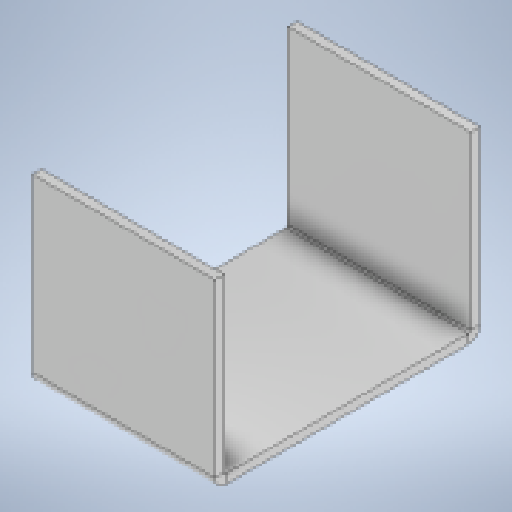
# Autodesk Inventor part: HWFrame
Saved by Autodesk Inventor 2025.2 (Build 292293000, 293)
## iProperties
Created: 2025-03-25
Part Number: HWFrame
Material: Aluminum 6061-AHC
Document SubType Name: Sheet Metal
Designer: User
Density: 2.7 g/cm^3
Sheet Metal Rule: Default_mm
Appearance: Aluminum - Dark
Author: User
Autodesk Inventor part; units mm, degrees
ref_plane "YZ Plane" through (0, 0, 0) normal (1, 0, 0) x (0, 1, 0)
ref_plane "XZ Plane" through (0, 0, 0) normal (0, 1, 0) x (-1, 0, 0)
ref_plane "XY Plane" through (0, 0, 0) normal (0, 0, 1) x (1, 0, 0)
sketch "Sketch1" plane through (0, 0, 0) normal (0, 1, 0) x (-1, 0, 0)
  line L0 (15, 20.25) -> (-15, 20.25)
  line L1 (-15, 20.25) -> (-15, -20.25)
  line L2 (-15, -20.25) -> (15, -20.25)
  line L3 (15, -20.25) -> (15, 20.25)
  line L4 (15, 20.25) -> (-15, -20.25) construction
  line L5 (-15, 20.25) -> (15, -20.25) construction
  point P0 (0, 0)
  dimension "d0" = 30
  dimension "d1" = 40.5
  measures "d0" distance of L1.end L2.end
  measures "d1" distance of L0.end L1.end
extrude "Plate1" add sketch "Sketch1" along normal blind 1.5
sketch "Sketch2" plane through (15, 0, 21.75) normal (0, 0, -1) x (-1, 0, 0)
  line L0 (30, 0) -> (0, 0)
  line L1 (0, 0) -> (0, 30)
  line L2 (0, 30) -> (30, 30)
  line L3 (30, 30) -> (30, 0)
  constraints: 8 end point
edge flange "Flange1" height 30 angle 90 thickness 1.5 bend radius 0.31 thickness toward (0, 0, -1) relief tear relief width 1.5 relief depth 0.75 corner gap 0.31 corner form 0 edges at (0, 1.5, 20.25) (0, 1.5, -20.25) wall of the first edge with corners at (-15, 0, 21.75) (15, 0, 21.75) (15, 30, 21.75) (-15, 30, 21.75)
bend "Bend1"
corner "Corner1"
sketch "Sketch3" plane through (-15, 30, 21.75) normal (0, 0, 1) x (1, 0, 0)
  circle A0 centre (22.525, -21) radius 0.7835 projected
  circle A1 centre (22.525, -5.9) radius 0.7835 projected
  circle A2 centre (7.475, -21) radius 0.7835 projected
  circle A3 centre (7.475, -5.9) radius 0.7835 projected
  ellipse E0 centre (22.952, 14.482) end of major axis (23.818, 15.348) minor radius 1 (24.07, 14.7056) -> (23.1756, 15.6) ccw projected
  line L0 (6.8244, 15.6) -> (23.1756, 15.6) projected
  ellipse E1 centre (7.048, 14.482) end of major axis (6.182, 15.348) minor radius 1 (6.8244, 15.6) -> (5.93, 14.7056) ccw projected
  line L1 (5.93, -21.6056) -> (5.93, 14.7056) projected
  ellipse E2 centre (7.048, -21.382) end of major axis (6.182, -22.248) minor radius 1 (5.93, -21.6056) -> (6.8244, -22.5) ccw projected
  line L2 (23.1756, -22.5) -> (6.8244, -22.5) projected
  ellipse E3 centre (22.952, -21.382) end of major axis (23.818, -22.248) minor radius 1 (23.1756, -22.5) -> (24.07, -21.6056) ccw projected
  line L3 (24.07, 14.7056) -> (24.07, -21.6056) projected
  circle A4 centre (7.475, -21) radius 0.7835 projected
  circle A5 centre (22.525, -21) radius 0.7835 projected
  circle A6 centre (7.475, -5.9) radius 0.7835 projected
  circle A7 centre (22.525, -5.9) radius 0.7835 projected
  circle A8 centre (7.475, 14.1) radius 0.7835 projected
  circle A9 centre (22.525, 14.1) radius 0.7835 projected
  circle A10 centre (15, 6.6) radius 6.4 projected
  point P0 (15, -30)
  constraints: 4 other
hole "Hole1" at (7.525, 24.1, 21.75) at (7.525, 9, 21.75) at (-7.525, 9, 21.75) at (-7.525, 24.1, 21.75) direction (0, 0, -1) diameter 2.1 depth 1.5
sketch "Sketch4" plane through (15, 30, -21.75) normal (0, 0, -1) x (-1, 0, 0)
  circle A0 centre (15, -20.82) radius 0.7835 projected
  circle A1 centre (8, -13.52) radius 0.7835 projected
  circle A2 centre (22, -13.52) radius 0.7835 projected
  circle A3 centre (7, -0.3) radius 0.7835 projected
  circle A4 centre (23, -0.3) radius 0.7835 projected
  line L0 (21.07, -22.22) -> (8.93, -22.22) projected
  line L1 (21.07, -22.22) -> (21.07, -21.5) projected
  arc A5 (23.07, -19.5) -> (21.07, -21.5) centre (23.07, -21.5) ccw projected
  line L2 (23.07, -19.5) -> (23.79, -19.5) projected
  line L3 (23.79, 12.6) -> (23.79, -19.5) projected
  line L4 (23.79, 12.6) -> (23.07, 12.6) projected
  arc A6 (21.07, 14.6) -> (23.07, 12.6) centre (23.07, 14.6) ccw projected
  line L5 (21.07, 14.6) -> (21.07, 15.32) projected
  line L6 (8.93, 15.32) -> (21.07, 15.32) projected
  line L7 (8.93, 15.32) -> (8.93, 14.6) projected
  arc A7 (6.93, 12.6) -> (8.93, 14.6) centre (6.93, 14.6) ccw projected
  line L8 (6.93, 12.6) -> (6.21, 12.6) projected
  line L9 (6.21, -19.5) -> (6.21, 12.6) projected
  line L10 (6.21, -19.5) -> (6.93, -19.5) projected
  arc A8 (8.93, -21.5) -> (6.93, -19.5) centre (6.93, -21.5) ccw projected
  line L11 (8.93, -21.5) -> (8.93, -22.22) projected
  circle A9 centre (15, 6.6) radius 6.4 projected
  point P0 (15, -30)
hole "Hole2" at (-7, 16.48, -21.75) at (7, 16.48, -21.75) at (0, 9.18, -21.75) direction (0, 0, 1) diameter 2.1 depth 1.5
equation "\"d18\" = Thickness"
equation "\"d25\" = Thickness"
equation "\"d2\" = Thickness"
equation "\"d3\" = BendReliefWidth"
equation "\"d4\" = BendReliefDepth"
equation "\"d5\" = MinimumRemnant"
equation "\"d6\" = TransitionRadius"
equation "\"d9\" = BendRadius"
equation "\"d10\" = CornerReliefSize"
equation "\"d11\" = GapSize"
equation "\"d12\" = JacobiRadiusSize"
equation "\"BendReliefWidth\" = Thickness"
equation "\"BendReliefDepth\" = 0.5 * Thickness"
equation "\"CornerReliefSize\" = 4 * Thickness"
equation "\"MinimumRemnant\" = 2 * Thickness"
equation "\"TransitionRadius\" = BendRadius"
equation "\"JacobiRadiusSize\" = BendRadius"
equation "\"GapSize\" = Thickness"
equation "\"Thickness\" = 1.5"
equation "\"BendRadius\" = 0.31"
body "Solid1"
